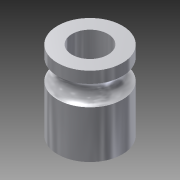
# Autodesk Inventor part: DriveGearMK8
Saved by Autodesk Inventor 2015 SP1 (Build 190203100, 203)
## iProperties
Created: 2014-12-06
Part Number: DriveGearMK8
Material: Aluminum 6061
Document SubType Name: Modeling
Designer: Jack
Density: 2.7 g/cm^3
Appearance: Aluminum - Flat
Mass: 1.12409 g
Surface Area: 5.86395 cm^2
Volume: 0.416331 cm^3
Vendor: RobotDigg
Author: Jack
Title: MK8 Drive Gear
Autodesk Inventor part; units mm, degrees
ref_plane "XZ Plane" through (0, 0, 0) normal (0, 1, 0) x (-1, 0, 0)
ref_plane "XY Plane" through (0, 0, 0) normal (0, 0, 1) x (1, 0, 0)
sketch "Sketch1" plane through (0, 0, 0) normal (0, 0, 1) x (1, 0, 0)
  circle A0 centre (0, 0) radius 4.5
  dimension "d0" = 9
  constraints: 1 centre point, 1 coincident
  measures "d0" diameter of A0
extrude "Extrusion1" add sketch "Sketch1" along normal blind 11
sketch "Sketch2" plane through (0, 0, 11) normal (0, 0, 1) x (1, 0, 0)
  circle A0 centre (0, 0) radius 4.5 projected
  circle A1 centre (0, 0) radius 2.5
  dimension "d3" = 5
  constraints: 1 centre point, 1 coincident
  measures "d3" diameter of A1
extrude "Extrusion2" cut sketch "Sketch2" against normal up to next contours A1
ref_plane "Work Plane1" through (-4.5, 0, 0) normal (1, 0, 0) x (0, 1, 0)
sketch "Sketch3" plane through (-4.5, 0, 0) normal (1, 0, 0) x (0, 1, 0)
  circle A0 centre (0, 3.5) radius 1.5
  point P0 (0, 0)
  dimension "d6" = 3.5
  dimension "d7" = 3
  constraints: 1 centre point, 1 vertical alignment
  measures "d6" distance of point (0, 0) A0.centre
  measures "d7" diameter of A0
extrude "Extrusion3" cut sketch "Sketch3" along normal up to next
thread "Thread1" size "M3x0.5" class "6H" standard "ANSI Metric M Profile" full length
sketch "Sketch4" plane through (0, 0, 0) normal (0, 1, 0) x (-1, 0, 0)
  line L0 (4.5, 0) -> (4.5, 11) projected
  circle A0 centre (5, 8) radius 1.5
  line L1 (0, 13.2) -> (0, -2.2) projected
  point P0 (0, 0)
  dimension "d12" = 3
  dimension "d13" = 0.5
  dimension "d14" = 8
  constraints: 1 centre point
  measures "d12" diameter of A0
  measures "d13" distance from line of L0 A0.centre
  measures "d14" vertical distance of L0.start A0.centre
revolve "Revolution1" cut sketch "Sketch4" angle 360 about axis through (0, 0, 11) along (0, 0, -1)
equation "\"d8\" = d7"
body "Solid1"
